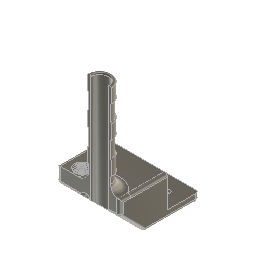
Cable Bowden Guide (Autodesk Fusion 360 design; units mm, degrees)
Autodesk Fusion 360 part; units mm, degrees
sketch "Sketch1" plane through (0, 0, 0) normal (0, 0, 1) x (1, 0, 0)
  line L0 (20, -25) -> (-20, -25)
  line L1 (-20, -25) -> (-20, 25)
  line L2 (-20, 25) -> (20, 25)
  line L3 (20, 25) -> (20, -25)
  line L4 (20, -25) -> (-20, 25) construction
  line L5 (-20, -25) -> (20, 25) construction
  line L6 (-20, 25) -> (20, 25)
  line L7 (20, 25) -> (20, 5)
  line L8 (20, 5) -> (-20, 5)
  line L9 (-20, 5) -> (-20, 25)
  arc A0 (12.5, -25) -> (1.5, -25) centre (7, -25) ccw
  arc A1 (14.5, -25) -> (-0.5, -25) centre (7, -25) ccw
  arc A2 (14, -25) -> (0, -25) centre (7, -25) ccw
  circle A3 centre (-10, -19) radius 1
  circle A4 centre (-10, -19) radius 4
  line L10 (-10, 25) -> (-10, 5) construction
  line L11 (-20, 15) -> (-10, 15) construction
  circle A5 centre (-10, 15) radius 1.75
  circle A6 centre (-10, 15) radius 3.25
  line L12 (20, -19) -> (-20, -19) construction
  line L13 (7, -25) -> (7, 5) construction
  line L14 (-10, -25) -> (-10, 5) construction
  line L15 (0, 25) -> (0, -25) construction
  circle A7 centre (10, 15) radius 3.25
  circle A8 centre (10, 15) radius 1.75
  dimension "d1" = 40
  dimension "d2" = 50
  dimension "d3" = 20
  dimension "d9" = 11
  dimension "d10" = 15
  dimension "d14" = 14
  dimension "d30" = 2
  dimension "d31" = 8
  dimension "d37" = 10
  dimension "d38" = 10
  dimension "d39" = 3.5
  dimension "d40" = 6.5
  dimension "d53" = 13
  dimension "d54" = 10
  dimension "d55" = 6
  constraint horizontal L0
  constraint perpendicular L0 L1
  constraint parallel L0 L2
  constraint parallel L1 L3
  constraint coincident L4 origin
  constraint coincident L5 origin
  constraint horizontal L6
  constraint vertical L7
  constraint horizontal L8
  constraint vertical L9
  constraint coincident L3 L7.end
  constraint coincident L0 A0.end
  constraint coincident L0 A0.start
  constraint coincident L0 A1.end
  constraint coincident L0 A1.start
  constraint coincident L0 A2.end
  constraint coincident L0 A2.start
  constraint concentric A3 A4
  constraint coincident L2 L10.start
  constraint coincident L8 L10.end
  constraint perpendicular L8 L10
  constraint coincident L1 L11.start
  constraint coincident L10 L11.end
  constraint perpendicular L10 L11
  constraint coincident L11.end A5.centre
  constraint concentric A5 A6
  constraint coincident L3 L12.start
  constraint coincident L1 L12.end
  constraint perpendicular L1 L12
  constraint coincident A3.centre L12
  constraint coincident L0 A0.centre
  constraint coincident A0.centre A1.centre
  constraint coincident L8 L13.end
  constraint perpendicular L8 L13
  constraint coincident L0 L14.start
  constraint perpendicular L8 L14
  constraint coincident A3.centre L14
  constraint midpoint L2 L15.start
  constraint midpoint L0 A2.end
  constraint symmetric A5 L15 A8
  constraint symmetric A6 L15 A7
  constraint coincident A0.centre L13
  measures "d1" distance of L1.end L2.end
  measures "d2" distance of L0.end L1.end
  measures "d3" distance of L1.end L8.end
  measures "d9" diameter of A0
  measures "d10" diameter of A1
  measures "d14" diameter of A2
  measures "d30" diameter of A3
  measures "d31" diameter of A4
  measures "d37" distance of L9 L10
  measures "d38" distance of L6 L11
  measures "d39" diameter of A5
  measures "d40" diameter of A6
  measures "d53" distance of L3 L13
  measures "d54" distance of L1 L14
  measures "d55" distance of L0 L12
extrude "Extrude1" add sketch "Sketch1" along normal blind 5 contours L0 L1 L3 L8 A1 | L0 A1 A2 | L1 L2 L3 L6 L7 L8 L9 | L0 A0 A2 | A4 | A6 | A7
extrude "Extrude2" add sketch "Sketch1" along normal blind 20 from surface at 5 contours L0 L1 L3 L8 A1 | L0 A1 A2 | L0 A0 A2 | A4
extrude "Extrude3" add sketch "Sketch1" along normal blind 10 from surface at 25 contours L0 A0 A2
extrude "Extrude4" add sketch "Sketch1" along normal blind 10 from surface at 35 contours L0 A1 A2 | L0 A0 A2
extrude "Extrude5" add sketch "Sketch1" along normal blind 10 from surface at 45 contours L0 A0 A2
extrude "Extrude6" add sketch "Sketch1" along normal blind 10 from surface at 55 contours L0 A1 A2 | L0 A0 A2
extrude "Extrude7" add sketch "Sketch1" along normal blind 10 from surface at 65 contours L0 A0 A2
extrude "Extrude8" add sketch "Sketch1" along normal blind 10 from surface at 75 contours L0 A1 A2 | L0 A0 A2
extrude "Extrude9" cut sketch "Sketch1" against normal blind 8 from surface at 25 contours A4
extrude "Extrude14" cut sketch "Sketch1" along normal blind 3 contours A6 | A7
extrude "Extrude15" add sketch "Sketch1" along normal blind 0.2 from surface at 3 contours A5 | A8
sketch "Sketch2" plane through (0, 0, 0) normal (0, 1, 0) x (1, 0, 0)
  line L0 (0, 0) -> (0, -25) construction
  line L1 (15.5518, -15) -> (-24.552, -15) construction
  line L2 (0, 0) -> (-20, 0) construction
  circle A0 centre (-2.1, -15) radius 1.75
  circle A1 centre (-2.1, -15) radius 3.25
  dimension "d58" = 15
  dimension "d59" = 3.5
  dimension "d60" = 6.5
  dimension "d77" = 2.1
  constraint coincident L0.start L2.start
  constraint vertical L0
  constraint perpendicular L0 L1
  constraint perpendicular L0 L2
  constraint concentric A0 A1
  constraint coincident L1 A0.centre
  measures "d58" distance of L1 L2
  measures "d59" diameter of A0
  measures "d60" diameter of A1
  measures "d77" distance of L0 A0.centre
extrude "Extrude11" cut sketch "Sketch2" against normal up to surface (30 mm away) from surface at 5 contours A0
extrude "Extrude12" cut sketch "Sketch2" along normal up to surface (27 mm away) from surface at -25
extrude "Extrude13" add sketch "Sketch2" along normal blind 0.2 from surface at 2 contours A0
thread "Thread1" "ISO Metric profile 10.0 M10x1 6H" major diameter 10.1472 minor diameter 9.0355 pitch 1 angle 60 modelled right hand crest width 0.2748 on face at (-6.0199, -19.3983, 22.3333) crest through (-5.4823, -19, 24.75)
chamfer "Chamfer1" distance 14 distance2 2 1 edges at (-10.9323, -18.6384, 0) measured on face at (-9.005, -19.0996, 5.6667)
chamfer "Chamfer2" distance 16 angle 45 2 edges at (16.25, -25, 0) (-9.25, -25, 0)
fillet "Fillet1" radius 6 1 edges at (7, -18, 25)
chamfer "Chamfer3" distance 0.5 angle 45 5 edges at (7, -17.5, 35) (7, -17.5, 45) (7, -17.5, 55) (7, -17.5, 65) (7, -17.5, 75)
fillet "Fillet2" radius 1 2 edges at (7, -19.5, 85) (7, -17.5, 85)
fillet "Fillet4" radius 2 14 edges at (-20, -10, 25) (-20, 8, 0) (-20, -17, 8) (-20, -25, 20.5) (-12.5962, -25, 16) (16.25, -25, 16) (20, -17, 8) (20, 8, 0) (0, -9, 0) (20, -10, 25) (20, -25, 20.5) (0, 25, 0) (20, 25, 2.5) (-20, 25, 2.5)
equation "d37 = d1 / 4"
equation "d38 = d3 / 2"
equation "d54 = d1 / 4"
